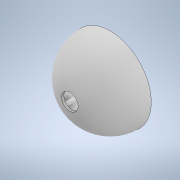
# Autodesk Inventor part: Eye
Saved by Autodesk Inventor 2022 (Build 260153000, 153)
## iProperties
Created: 2021-11-09
Part Number: Eye
Material: Generic
Document SubType Name: Modeling
Designer: Juan
Density: 1 g/cm^3
Appearance: Default
Author: Juan
Autodesk Inventor part; units mm, degrees
ref_plane "YZ Plane" through (0, 0, 0) normal (1, 0, 0) x (0, 1, 0)
ref_plane "XZ Plane" through (0, 0, 0) normal (0, 1, 0) x (-1, 0, 0)
sketch "Sketch4" plane through (0, 0, 0) normal (1, 0, 0) x (0, 1, 0)
  circle A0 centre (0, 0) radius 27.5
  circle A1 centre (0, 0) radius 26
  line L0 (0, 0) -> (0, 27.5)
  line L1 (0, 27.5) -> (5.5, 27.5)
  line L2 (5.5, 27.5) -> (5.5, 25.4116)
  line L3 (0, 27.5) -> (-5.5, 27.5)
  line L4 (-5.5, 27.5) -> (-5.5, 25.4116)
  line L5 (27.5, 0) -> (-27.5, 0)
  point P0 (26, 0)
  point P1 (5.5, 26.9444)
  dimension "d20" = 55
  dimension "d21" = 52
  dimension "d22" = 5.5
  dimension "d23" = 5.5
  constraints: 12 end point, 5 point on circle, 3 perpendicular, 2 centre point, 2 coincident, 1 horizontal, 1 point on line, 1 tangent, 1 vertical
  measures "d20" diameter of A0
  measures "d21" diameter of A1
  measures "d22" distance of L0.end L1.end
  measures "d23" distance of L0.end L3.end
revolve "Revolution2" add sketch "Sketch4" angle 360 about axis through (0, 0, 0) along (0, 0, 1) contours L5 A1 L2 A0
ref_plane "Work Plane1" through (0, 0, 5) normal (0, 0, -1) x (-1, 0, 0)
sketch "Sketch5" plane through (0, 0, 5) normal (0, 0, -1) x (-1, 0, 0)
  line L0 (-12, -12.25) -> (12, -12.25)
  line L1 (12, -12.25) -> (12, 12.25)
  line L2 (12, 12.25) -> (-12, 12.25)
  line L3 (-12, 12.25) -> (-12, -12.25)
  line L4 (-12, -12.25) -> (12, 12.25) construction
  line L5 (12, -12.25) -> (-12, 12.25) construction
  circle A0 centre (-12, 12.25) radius 1.25
  circle A1 centre (12, 12.25) radius 1.25
  circle A2 centre (12, -12.25) radius 1.25
  circle A3 centre (-12, -12.25) radius 1.25
  point P0 (0, 0)
  dimension "d26" = 24
  dimension "d27" = 24.5
  dimension "d28" = 2.5
  constraints: 12 end point, 4 centre point, 4 coincident, 3 equal radius, 2 midpoint, 2 parallel, 1 horizontal, 1 perpendicular
  measures "d26" distance of L2.end L1.end
  measures "d27" distance of L1.end L0.end
  measures "d28" diameter of A0
extrude "Extrusion3" add sketch "Sketch5" against normal up to surface contours L3 A3 L0 | L0 A3 L3 | A2 L1 L0 | L0 L1 A2 | A0 L2 L3 | L3 L2 A0 | A1 L2 L1 | L1 L2 A1
sketch "Sketch6" plane through (0, 0, 0) normal (0, 0, -1) x (-1, 0, 0)
  circle A0 centre (0, 0) radius 26 projected
  line L0 (-26, 0) -> (-26.75, 0)
  line L1 (-26.75, 0) -> (-26.75, 3)
  line L2 (-26.75, 3) -> (26.75, 3)
  line L3 (26.75, 3) -> (26.75, -3)
  line L4 (26.75, -3) -> (-26.75, -3)
  line L5 (-26.75, -3) -> (-26.75, 3)
  line L6 (0, 26) -> (0, 26.75)
  line L7 (0, 26.75) -> (3, 26.75)
  line L8 (3, 26.75) -> (-3, 26.75)
  line L9 (-3, 26.75) -> (-3, -26.75)
  line L10 (-3, -26.75) -> (3, -26.75)
  line L11 (3, -26.75) -> (3, 26.75)
  point P0 (-3, 3)
  point P1 (-25.8263, 3)
  point P2 (-25.8263, -3)
  point P3 (25.8263, -3)
  point P4 (25.8263, 3)
  point P5 (3, 3)
  point P6 (3, 25.8263)
  point P7 (-3, 25.8263)
  point P8 (3, -25.8263)
  point P9 (-3, -25.8263)
  point P10 (3, -3)
  point P11 (-3, -3)
  dimension "d31" = 0.75
  dimension "d32" = 3
  dimension "d33" = 53.5
  dimension "d34" = 6
  dimension "d35" = 0.75
  dimension "d36" = 3
  dimension "d37" = 6
  dimension "d38" = 53.5
  constraints: 24 end point, 4 parallel, 4 perpendicular, 3 horizontal, 2 point on circle, 1 vertical
  measures "d31" distance of L0.start L0.end
  measures "d32" distance of L0.end L1.end
  measures "d33" distance of L3.end L4.end
  measures "d34" distance of L2.end L3.end
  measures "d35" distance of L6.start L6.end
  measures "d36" distance of L6.end L7.end
  measures "d37" distance of L10.end L9.end
  measures "d38" distance of L9.end L8.end
extrude "Extrusion4" add sketch "Sketch6" against normal blind 3 contours A0 L4 L11 L2 | L11 L2 L9 A0 | L11 L4 L9 L2 | L9 L4 A0 L2
sketch "Sketch7" plane through (0, 0, 0) normal (0, 0, -1) x (-1, 0, 0)
  line L0 (0, 0) -> (22.5, 0)
  line L1 (0, 0) -> (-22.5, 0)
  line L2 (0, 0) -> (0, 22.5)
  circle A0 centre (0, 22.5) radius 1.6
  circle A1 centre (-22.5, 0) radius 1.6
  circle A2 centre (22.5, 0) radius 1.6
  dimension "d41" = 22.5
  dimension "d42" = 22.5
  dimension "d43" = 22.5
  dimension "d44" = 3.2
  dimension "d45" = 3.2
  dimension "d46" = 3.2
  constraints: 6 end point, 3 centre point, 3 coincident, 2 horizontal, 1 vertical
  measures "d41" distance of L0.start L0.end
  measures "d42" distance of L0.start L1.end
  measures "d43" distance of L0.start L2.end
  measures "d44" diameter of A0
  measures "d45" diameter of A1
  measures "d46" diameter of A2
extrude "Extrusion5" cut sketch "Sketch7" against normal up to surface
sketch "Sketch8" plane through (0, 0, 0) normal (0, 0, -1) x (-1, 0, 0)
  circle A0 centre (0, 0) radius 2.5
  circle A1 centre (0, 0) radius 2
  line L0 (2.5, -0.7) -> (-2.5, -0.7)
  line L1 (-2.5, -0.7) -> (-2.5, 0.7)
  line L2 (-2.5, 0.7) -> (2.5, 0.7)
  line L3 (2.5, 0.7) -> (2.5, -0.7)
  line L4 (2.5, -0.7) -> (-2.5, 0.7) construction
  line L5 (-2.5, -0.7) -> (2.5, 0.7) construction
  line L6 (-0.7, -2.5) -> (-0.7, 2.5)
  line L7 (-0.7, 2.5) -> (0.7, 2.5)
  line L8 (0.7, 2.5) -> (0.7, -2.5)
  line L9 (0.7, -2.5) -> (-0.7, -2.5)
  line L10 (-0.7, -2.5) -> (0.7, 2.5) construction
  line L11 (-0.7, 2.5) -> (0.7, -2.5) construction
  point P0 (-0.7, 1.8735)
  point P1 (-1.8735, 0.7)
  point P2 (-2.4, 0.7)
  point P3 (-2.4, -0.7)
  point P4 (-1.8735, -0.7)
  point P5 (-0.7, -1.8735)
  point P6 (-0.7, -2.4)
  point P7 (0.7, -2.4)
  point P8 (0.7, -1.8735)
  point P9 (1.8735, -0.7)
  point P10 (2.4, -0.7)
  point P11 (2.4, 0.7)
  point P12 (1.8735, 0.7)
  point P13 (0.7, 1.8735)
  point P14 (0.7, 2.4)
  point P15 (-0.7, 2.4)
  dimension "d49" = 5
  dimension "d50" = 4
  dimension "d51" = 1.4
  dimension "d52" = 1.4
  constraints: 24 end point, 4 midpoint, 4 parallel, 2 centre point, 2 coincident, 2 perpendicular, 1 horizontal, 1 vertical
  measures "d49" diameter of A0
  measures "d50" diameter of A1
  measures "d51" distance of L0.end L1.end
  measures "d52" distance of L6.end L7.end
extrude "Extrusion6" cut sketch "Sketch8" against normal blind 10 contours A0 L0 A1 L2 | L8 A1 L6 A0 | L2 L8 A1 | A1 L0 L8 L2 | A0 L6 A1 L8 | A1 L8 L0 | L8 L2 L6 A1 | L8 L0 L6 L2 | A1 L6 L0 L8 | L6 L2 A1 | L6 L0 A1 L2 | A1 L0 L6 | L2 A1 L0 A0
equation "\"d39\" = d32"
body "Solid2"
